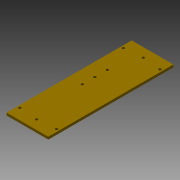
# Autodesk Inventor part: Paint Platforml
Saved by Autodesk Inventor 2013 SP2 (Build 170200200, 200)
## iProperties
Created: 2017-01-25
Part Number: Paint Platforml
Material: Generic
Document SubType Name: Modeling
Designer: Herman de Vries
Density: 1 g/cm^3
Mass: 14.7188 g
Surface Area: 110.688 cm^2
Volume: 14.7188 cm^3
Author: Herman de Vries
Autodesk Inventor part; units mm, degrees
ref_plane "YZ Plane" through (0, 0, 0) normal (1, 0, 0) x (0, 1, 0)
ref_plane "XZ Plane" through (0, 0, 0) normal (0, 1, 0) x (-1, 0, 0)
ref_plane "XY Plane" through (0, 0, 0) normal (0, 0, 1) x (1, 0, 0)
sketch "Sketch1" plane through (0, 0, 0) normal (0, 1, 0) x (-1, 0, 0)
  line L0 (0, 0) -> (50, 0)
  line L1 (50, 0) -> (50, 3)
  line L2 (50, 3) -> (0, 3)
  line L3 (0, 3) -> (0, 0)
  dimension "d0" = 50
  dimension "d1" = 3
  constraints: 8 end point, 2 parallel, 1 horizontal, 1 perpendicular
  measures "d0" distance of L2.end L1.end
  measures "d1" distance of L1.end L0.end
extrude "Extrusion1" add sketch "Sketch1" along normal blind 150
sketch "Sketch3" plane through (0, 0, 0) normal (0, 0, -1) x (-1, 0, 0)
  circle A0 centre (3, 13) radius 1.6 projected
  circle A1 centre (25, 11) radius 1.6 projected
  circle A2 centre (47, 13) radius 1.6 projected
  circle A3 centre (3, 137) radius 1.6 projected
  circle A4 centre (25, 139) radius 1.6 projected
  circle A5 centre (47, 137) radius 1.6 projected
  circle A6 centre (34, 91.5) radius 1.6 projected
  circle A7 centre (34, 106.5) radius 1.6
  circle A8 centre (34, 76.5) radius 1.6
  circle A9 centre (34, 121.5) radius 1.6 projected
  dimension "d18" = 3.2
  dimension "d19" = 3.2
  dimension "d21" = 15
  constraints: 2 centre point, 2 vertical alignment
  measures "d18" diameter of A7
  measures "d19" diameter of A8
  measures "d21" distance of A8.centre A6.centre
extrude "Extrusion3" cut sketch "Sketch3" against normal blind 10
equation "\"d21\" = d20"
equation "\"d20\" = 15"
body "Solid1"
